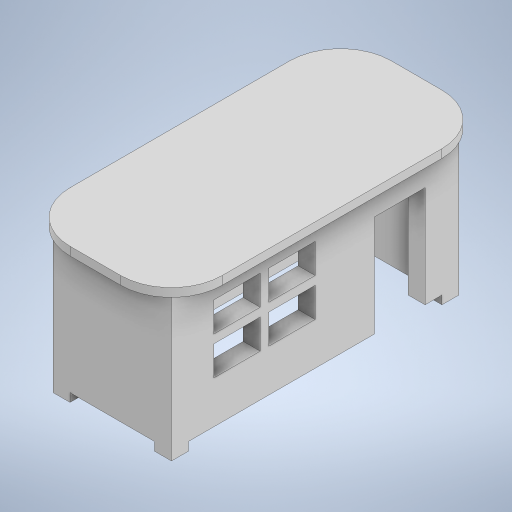
# Autodesk Inventor part: huis
Saved by Autodesk Inventor 2023 (Build 270158000, 158)
## iProperties
Created: 2023-06-06
Part Number: huis
Material: Generic
Document SubType Name: Modeling
Designer: Prestige
Density: 1 g/cm^3
Appearance: Default
Author: Prestige
Autodesk Inventor part; units mm, degrees
ref_plane "YZ Plane" through (0, 0, 0) normal (1, 0, 0) x (0, 1, 0)
ref_plane "XZ Plane" through (0, 0, 0) normal (0, 1, 0) x (-1, 0, 0)
ref_plane "XY Plane" through (0, 0, 0) normal (0, 0, 1) x (1, 0, 0)
sketch "Sketch1" plane through (0, 0, 0) normal (0, 1, 0) x (-1, 0, 0)
  line L0 (0, 0) -> (10, 0)
  line L1 (10, 0) -> (10, -10)
  line L2 (10, -10) -> (0, -10)
  line L3 (0, -10) -> (0, 0)
  line L4 (10, -160) -> (0, -160)
  line L5 (0, -160) -> (0, -170)
  line L6 (0, -170) -> (10, -170)
  line L7 (10, -170) -> (10, -160)
  line L8 (60, -170) -> (70, -170)
  line L9 (70, -170) -> (70, -160)
  line L10 (70, -160) -> (60, -160)
  line L11 (60, -160) -> (60, -170)
  line L12 (70, -10) -> (60, -10)
  line L13 (60, -10) -> (60, 0)
  line L14 (60, 0) -> (70, 0)
  line L15 (70, 0) -> (70, -10)
  point P0 (10, -5)
  dimension "d0" = 10
  dimension "d1" = 10
  dimension "d2" = 10
  dimension "d3" = 10
  dimension "d4" = 10
  dimension "d5" = 10
  dimension "d6" = 150
  dimension "d7" = 50
  constraints: 32 end point, 8 parallel, 7 point on line, 4 horizontal, 4 perpendicular, 1 midpoint
  measures "d0" distance of L12.start L12.end
  measures "d1" distance of L14.end L12.start
  measures "d2" distance of L9.end L10.end
  measures "d3" distance of L8.end L9.end
  measures "d4" distance of L5.end L6.end
  measures "d5" distance of L0.end L1.end
  measures "d6" distance between parallel lines of L12 L10
  measures "d7" distance from line of L13 point (10, -5)
extrude "Extrusion1" add sketch "Sketch1" along normal blind 5
sketch "Sketch2" plane through (0, 5, 0) normal (0, 1, 0) x (1, 0, 0)
  line L0 (-70, 0) -> (-60, 0) projected
  line L1 (-70, 0) -> (-60, 0)
  line L2 (-60, 0) -> (-60, 170)
  line L3 (-60, 170) -> (-70, 170)
  line L4 (-70, 170) -> (-70, 0)
  line L5 (-10, 160) -> (0, 160) projected
  line L6 (-60, 170) -> (0, 170)
  line L7 (0, 170) -> (0, 160)
  line L8 (0, 160) -> (-60, 160)
  line L9 (-60, 160) -> (-60, 170)
  line L10 (-10, 0) -> (0, 0) projected
  line L11 (-10, 160) -> (0, 160)
  line L12 (0, 160) -> (0, 0)
  line L13 (0, 0) -> (-10, 0)
  line L14 (-10, 0) -> (-10, 160)
  line L15 (-10, 0) -> (-60, 0)
  line L16 (-60, 0) -> (-60, 10)
  line L17 (-60, 10) -> (-10, 10)
  line L18 (-10, 10) -> (-10, 0)
  point P0 (0, 160)
  constraints: 32 end point, 8 parallel, 4 horizontal, 4 perpendicular
extrude "Extrusion2" add sketch "Sketch2" along normal blind 80 contours L4 L3 L2 L0 | L2 L17 L14 L15 | L14 L5 L12 L10 | L6 L7 L5 L8 L2
sketch "Sketch3" plane through (0, 85, 0) normal (0, 1, 0) x (1, 0, 0)
  line L0 (-80, -10) -> (10, -10)
  line L1 (10, -10) -> (10, 180)
  line L2 (10, 180) -> (-80, 180)
  line L3 (-80, 180) -> (-80, -10)
  line L4 (-70, 170) -> (-70, 0) projected
  line L5 (0, 170) -> (-70, 170) projected
  line L6 (0, 0) -> (0, 170) projected
  line L7 (-70, 0) -> (0, 0) projected
  point P0 (-35, -10)
  dimension "d12" = 10
  dimension "d13" = 10
  dimension "d14" = 10
  dimension "d15" = 10
  constraints: 8 end point, 2 parallel, 1 horizontal, 1 midpoint, 1 perpendicular
  measures "d12" distance between parallel lines of L3 L4
  measures "d13" distance between parallel lines of L2 L5
  measures "d14" distance between parallel lines of L6 L1
  measures "d15" distance from line of L7 point (-35, -10)
extrude "Extrusion3" add sketch "Sketch3" along normal blind 5 contours L3 L2 L1 L0 | L5 L6 L7 L4
fillet "Fillet1" radius 30 4 edges at (10, 87.5, 10) (-80, 87.5, 10) (-80, 87.5, -180) (10, 87.5, -180)
sketch "Sketch4" plane through (0, 0, 0) normal (1, 0, 0) x (0, 0, -1)
  line L0 (150, 5) -> (120, 5)
  line L1 (120, 5) -> (120, 65)
  line L2 (120, 65) -> (150, 65)
  line L3 (150, 65) -> (150, 5)
  line L4 (25, 70) -> (85, 70)
  line L5 (85, 70) -> (85, 30)
  line L6 (85, 30) -> (25, 30)
  line L7 (25, 30) -> (25, 70)
  line L8 (0, 0) -> (0, 85) projected
  line L9 (170, 0) -> (170, 85) projected
  line L10 (10, 5) -> (160, 5) projected
  line L11 (20, 85) -> (150, 85) projected
  line L12 (52.5, 70) -> (57.5, 70)
  line L13 (57.5, 70) -> (57.5, 30)
  line L14 (57.5, 30) -> (52.5, 30)
  line L15 (52.5, 30) -> (52.5, 70)
  line L16 (85, 52.5) -> (25, 52.5)
  line L17 (25, 52.5) -> (25, 47.5)
  line L18 (25, 47.5) -> (85, 47.5)
  line L19 (85, 47.5) -> (85, 52.5)
  point P0 (52.5, 52.5)
  point P1 (52.5, 47.5)
  point P2 (57.5, 47.5)
  point P3 (57.5, 52.5)
  dimension "d19" = 60
  dimension "d20" = 30
  dimension "d21" = 40
  dimension "d22" = 60
  dimension "d23" = 25
  dimension "d24" = 20
  dimension "d25" = 0
  dimension "d26" = 15
  dimension "d27" = 5
  dimension "d28" = 5
  dimension "d29" = 17.5
  dimension "d30" = 27.5
  constraints: 32 end point, 8 parallel, 4 horizontal, 4 perpendicular, 4 point on line
  measures "d19" distance of L2.end L0.start
  measures "d20" distance of L1.end L2.end
  measures "d21" distance of L4.end L5.end
  measures "d22" distance of L4.start L4.end
  measures "d23" distance between parallel lines of L8 L7
  measures "d24" distance between parallel lines of L9 L3
  measures "d25" distance between parallel lines of L10 L0
  measures "d26" distance between parallel lines of L11 L4
  measures "d27" distance between parallel lines of L15 L13
  measures "d28" distance between parallel lines of L18 L16
  measures "d29" distance between parallel lines of L4 L16
  measures "d30" distance between parallel lines of L5 L13
extrude "Extrusion4" cut sketch "Sketch4" against normal blind 10 contours L0 L1 L2 L3 | L4 L15 L16 L7 | L4 L5 L16 L13 | L18 L15 L6 L7 | L18 L5 L6 L13
body "Solid1"
